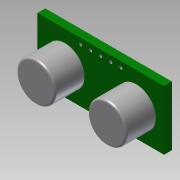
# Autodesk Inventor part: srf10
Saved by Autodesk Inventor 2015 SP1 (Build 190203100, 203)
## iProperties
Created: 2015-01-27
Part Number: srf10
Material: Generic
Document SubType Name: Modeling
Designer: Rafi Kurnia Putra
Density: 1 g/cm^3
Appearance: Default
Author: Rafi Kurnia Putra
Autodesk Inventor part; units mm, degrees
ref_plane "YZ Plane" through (0, 0, 0) normal (1, 0, 0) x (0, 1, 0)
ref_plane "XZ Plane" through (0, 0, 0) normal (0, 1, 0) x (-1, 0, 0)
ref_plane "XY Plane" through (0, 0, 0) normal (0, 0, 1) x (1, 0, 0)
sketch "Sketch1" plane through (0, 0, 0) normal (0, 0, 1) x (1, 0, 0)
  line L0 (-16, 7.5) -> (16, 7.5)
  line L1 (16, 7.5) -> (16, -7.5)
  line L2 (16, -7.5) -> (-16, -7.5)
  line L3 (-16, -7.5) -> (-16, 7.5)
  line L4 (-16, 0) -> (-16, 7.5)
  line L5 (-16, 7.5) -> (0, 7.5)
  point P0 (0, 0)
  dimension "d0" = 32
  dimension "d1" = 15
  constraints: 12 end point, 2 parallel, 1 horizontal, 1 perpendicular
  measures "d0" distance of L1.end L2.end
  measures "d1" distance of L0.end L1.end
extrude "Extrusion1" add sketch "Sketch1" against normal blind 2
sketch "Sketch2" plane through (0, 0, 0) normal (0, 0, 1) x (1, 0, 0)
  line L0 (-16, 7.5) -> (16, 7.5) projected
  line L1 (-16, -7.5) -> (-16, 7.5) projected
  line L2 (16, -7.5) -> (-16, -7.5) projected
  line L3 (16, 7.5) -> (16, -7.5) projected
  circle A0 centre (-9, -0.5) radius 4.9
  circle A1 centre (9, -0.5) radius 4.9
  circle A2 centre (0, 6.06) radius 0.4
  circle A3 centre (-2.54, 6.06) radius 0.4
  circle A4 centre (-5.08, 6.06) radius 0.4
  line L4 (0, 0) -> (0, 3) construction
  line L5 (0, 3) -> (0, 0) construction
  line L6 (16, 7.5) -> (-16, 7.5)
  circle A5 centre (2.54, 6.06) radius 0.4
  circle A6 centre (5.08, 6.06) radius 0.4
  point P0 (8.9861, 0.5)
  dimension "d8" = 9.8
  dimension "d11" = 32
  dimension "d12" = 15
  dimension "d16" = 8
  dimension "d17" = 9.8
  dimension "d19" = 9
  dimension "d20" = 9
  dimension "d24" = 0.8
  dimension "d25" = 1.44
  dimension "d26" = 0.8
  dimension "d27" = 2.54
  dimension "d28" = 0.8
  dimension "d29" = 2.54
  constraints: 7 centre point, 6 end point, 4 symmetric about line, 1 collinear, 1 horizontal alignment, 2 other
  measures "d8" diameter of A0
  measures "d11" distance of L0.start L0.end
  measures "d12" distance of L0.end L2.start
  measures "d16" distance from line of A0.centre L0
  measures "d17" diameter of A1
  measures "d19" horizontal distance of L4.start A0.centre
  measures "d20" horizontal distance of L4.start A1.centre
  measures "d24" diameter of A2
  measures "d25" distance from line of A2.centre L0
  measures "d26" diameter of A3
  measures "d27" distance of A2.centre A3.centre
  measures "d28" diameter of A4
  measures "d29" distance of A3.centre A4.centre
extrude "Extrusion3" add sketch "Sketch2" along normal blind 7.4 contours A0 | A1
fillet "Fillet2" radius 0.5 2 edges at (-13.9, -0.5, 7.4) (4.1, -0.5, 7.4)
extrude "Extrusion4" cut sketch "Sketch2" against normal up to next contours A2 | A3 | A4 | A5 | A6
body "Solid1"
